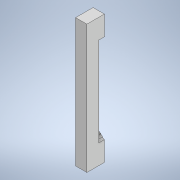
# Autodesk Inventor part: Base Drawing
Saved by Autodesk Inventor 2020 (Build 240168000, 168)
## iProperties
Created: 2020-04-06
Part Number: Base Drawing
Material: Generic
Document SubType Name: Modeling
Designer: Thomas J H Dodd
Density: 1 g/cm^3
Appearance: Default
Author: Thomas J H Dodd
Autodesk Inventor part; units mm, degrees
ref_plane "YZ Plane" through (0, 0, 0) normal (1, 0, 0) x (0, 1, 0)
ref_plane "XZ Plane" through (0, 0, 0) normal (0, 1, 0) x (-1, 0, 0)
ref_plane "XY Plane" through (0, 0, 0) normal (0, 0, 1) x (1, 0, 0)
sketch "Sketch1" plane through (0, 0, 0) normal (0, 1, 0) x (-1, 0, 0)
  line L0 (0, 0) -> (0, -300)
  line L1 (0, -300) -> (-115, -300)
  line L2 (-115, -300) -> (-115, -355)
  line L3 (-115, -355) -> (-230, -355)
  line L4 (-230, -355) -> (-345, -355) construction
  line L5 (0, 0) -> (-345, 0)
  line L6 (-345, 0) -> (-345, -240)
  line L7 (-270, -300) -> (-270, -315)
  line L8 (-345, -240) -> (-270, -300) construction
  line L9 (-307.5, -270) -> (-270, -300) construction
  line L10 (-307.5, -270) -> (-345, -240) construction
  arc A0 (-307.5, -270) -> (-270, -300) centre (-260.624645, -249.843306) ccw
  arc A1 (-307.5, -270) -> (-345, -240) centre (-353.647258, -289.246573) ccw
  arc A2 (-230, -355) -> (-270, -315) centre (-270.80177, -355.80177) ccw
  point P0 (-288.75, -285)
  point P1 (-326.25, -255)
  dimension "d0" = 300
  dimension "d1" = 115
  dimension "d2" = 55
  dimension "d3" = 115
  dimension "d4" = 115
  dimension "d5" = 345
  dimension "d7" = 15
  dimension "d8" = 155
  dimension "d9" = 40
  dimension "d13" = 50
  dimension "d14" = 50
  dimension "d16" = 62.5
  dimension "d19" = 60
  constraints: 22 end point, 6 point on circle, 3 centre point, 3 horizontal, 3 midpoint, 3 perpendicular, 2 vertical, 1 collinear
  measures "d0" distance of L0.start L0.end
  measures "d1" distance of L0.end L1.end
  measures "d2" distance of L1.end L2.end
  measures "d3" distance of L2.end L3.end
  measures "d4" distance of L3.end L4.end
  measures "d5" distance of L0.start L5.end
  measures "d7" distance of L7.start L7.end
  measures "d8" distance between parallel lines of L7 L2
  measures "d9" distance from line of L3 L7.end
  measures "d14" radius of A1
  measures "d19" vertical distance of L7.start L6.end
extrude "Extrusion1" add sketch "Sketch1" along normal blind 299
sketch "Sketch2" plane through (0, 299, 0) normal (0, 1, 0) x (1, 0, 0)
  line L0 (230, 355) -> (115, 355)
  line L1 (115, 355) -> (115, 300)
  line L2 (115, 300) -> (0, 300)
  line L3 (0, 300) -> (0, 0)
  line L4 (0, 0) -> (345, 0)
  line L5 (345, 0) -> (345, 240)
  arc A0 (307.5, 270) -> (345, 240) centre (353.647258, 289.246573) ccw
  arc A1 (307.5, 270) -> (270, 300) centre (260.624645, 249.843306) ccw
  line L6 (270, 300) -> (270, 315)
  arc A2 (230, 355) -> (270, 315) centre (270.80177, 355.80177) ccw
extrude "Extrusion2" add sketch "Sketch2" along normal blind 1281
sketch "Sketch3" plane through (0, 0, 0) normal (0, -1, 0) x (1, 0, 0)
  line L0 (230, -355) -> (115, -355) projected
  line L1 (115, -355) -> (115, -300) projected
  line L2 (115, -300) -> (0, -300) projected
  line L3 (0, -300) -> (0, 0) projected
  line L4 (0, 0) -> (345, 0) projected
  line L5 (345, 0) -> (345, -240) projected
  line L6 (230, -355) -> (345, -355)
  line L7 (345, -355) -> (345, -240)
  constraints: 4 end point, 1 horizontal, 1 perpendicular
extrude "Extrusion3" add sketch "Sketch3" along normal blind 515
sketch "Sketch4" plane through (0, 1580, 0) normal (0, 1, 0) x (1, 0, 0)
  line L0 (345, 0) -> (345, 240) projected
  line L1 (0, 0) -> (345, 0) projected
  line L2 (0, 300) -> (0, 0) projected
  line L3 (115, 300) -> (0, 300) projected
  line L4 (115, 355) -> (115, 300) projected
  line L5 (345, 355) -> (345, 240) projected
  line L6 (345, 240) -> (345, 355)
  line L7 (345, 355) -> (115, 355)
  constraints: 4 end point, 1 collinear, 1 perpendicular
extrude "Extrusion4" add sketch "Sketch4" along normal blind 515
sketch "Sketch5" plane through (0, 1580, 0) normal (0, -1, 0) x (1, 0, 0)
  arc A0 (270, -315) -> (230, -355) centre (270.80177, -355.80177) ccw
  line L0 (345, -355) -> (230, -355)
  line L1 (345, -240) -> (345, -355)
  arc A1 (345, -240) -> (307.5, -270) centre (353.647258, -289.246573) ccw
  arc A2 (270, -300) -> (307.5, -270) centre (260.624645, -249.843306) ccw
  line L2 (270, -300) -> (270, -315)
  line L3 (424.37671, -355) -> (-70.729452, -355)
  point P0 (0, 0)
revolve "Revolution1" cut sketch "Sketch5" angle 360 about axis through (345, 1580, -355) along (-1, 0, 0)
sketch "Sketch6" plane through (0, 0, 0) normal (0, 1, 0) x (1, 0, 0)
  arc A0 (307.5, 270) -> (345, 240) centre (353.647258, 289.246573) ccw
  line L0 (345, 355) -> (345, 240)
  line L1 (230, 355) -> (345, 355)
  arc A1 (230, 355) -> (270, 315) centre (270.80177, 355.80177) ccw
  line L2 (270, 300) -> (270, 315)
  arc A2 (307.5, 270) -> (270, 300) centre (260.624645, 249.843306) ccw
  line L3 (-70.729452, 355) -> (424.37671, 355)
  point P0 (0, 0)
revolve "Revolution2" cut sketch "Sketch6" angle 360 about axis through (115, 0, -355) along (1, 0, 0)
sketch "Sketch12" plane through (345, -515, -355) normal (0, 0, -1) x (-1, 0, 0)
  arc A0 (0, 400) -> (37.5, 430) centre (-8.647258, 449.246573) ccw
  arc A1 (75, 460) -> (37.5, 430) centre (84.375355, 409.843306) ccw
  line L0 (75, 475) -> (75, 460)
  arc A2 (75, 475) -> (115, 515) centre (74.19823, 515.80177) ccw
  line L1 (0, 515) -> (37.5, 515)
  line L2 (75, 515) -> (37.5, 515)
  line L3 (75, 515) -> (115, 515)
  line L4 (0, 400) -> (0, 515)
  point P0 (345, 515)
extrude "Extrusion10" cut sketch "Sketch12" against normal blind 115
sketch "Sketch13" plane through (345, -515, -355) normal (0, 0, -1) x (-1, 0, 0)
  arc A0 (115, 2095) -> (75, 2135) centre (74.19823, 2094.19823) ccw
  line L0 (75, 2150) -> (75, 2135)
  arc A1 (37.5, 2180) -> (75, 2150) centre (84.375355, 2200.156694) ccw
  arc A2 (37.5, 2180) -> (0, 2210) centre (-8.647258, 2160.753427) ccw
  line L1 (0, 2095) -> (0, 2210)
  line L2 (0, 2095) -> (37.5, 2095)
  line L3 (75, 2095) -> (37.5, 2095)
  line L4 (75, 2095) -> (115, 2095)
  point P0 (345, 515)
extrude "Extrusion11" cut sketch "Sketch13" against normal blind 115
sketch "Sketch14" plane through (230, 0, -240) normal (0, -1, 0) x (1, 0, 0)
  arc A0 (40, -75) -> (0, -115) centre (40.80177, -115.80177) ccw
  line L0 (40, -60) -> (40, -75)
  arc A1 (40, -60) -> (77.5, -30) centre (30.624645, -9.843306) ccw
  arc A2 (115, 0) -> (77.5, -30) centre (123.647258, -49.246573) ccw
  line L1 (115, 0) -> (0, 0)
  line L2 (0, -115) -> (0, 0)
  point P0 (-230, 240)
extrude "Extrusion12" add sketch "Sketch14" along normal up to next
sketch "Sketch15" plane through (230, 1580, -240) normal (0, 1, 0) x (1, 0, 0)
  arc A0 (77.5, 30) -> (115, 0) centre (123.647258, 49.246573) ccw
  arc A1 (77.5, 30) -> (40, 60) centre (30.624645, 9.843306) ccw
  line L0 (40, 75) -> (40, 60)
  arc A2 (0, 115) -> (40, 75) centre (40.80177, 115.80177) ccw
  line L1 (0, 115) -> (0, 0)
  line L2 (0, 0) -> (115, 0)
  point P0 (-230, -240)
extrude "Extrusion13" add sketch "Sketch15" along normal up to next
sketch "Sketch16" plane through (0, -515, 0) normal (0, -1, 0) x (1, 0, 0)
  line L0 (0, -300) -> (115, -300) projected
  line L1 (0, 0) -> (0, -300) projected
  line L2 (0, 0) -> (115, 0)
  line L3 (115, 0) -> (115, -300)
  constraints: 4 end point, 1 perpendicular
extrude "Extrusion14" cut sketch "Sketch16" against normal through all
body "Solid1"
